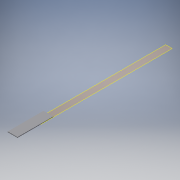
# Autodesk Inventor part: Part1
Saved by Autodesk Inventor 2016 (Build 200138000, 138)
## iProperties
Created: 2017-06-06
Part Number: Part1
Material: Generic
Document SubType Name: Modeling
Designer: m228540
Density: 1 g/cm^3
Appearance: Default
Author: m228540
Autodesk Inventor part; units mm, degrees
ref_plane "YZ Plane" through (0, 0, 0) normal (1, 0, 0) x (0, 1, 0)
ref_plane "XZ Plane" through (0, 0, 0) normal (0, 1, 0) x (-1, 0, 0)
ref_plane "XY Plane" through (0, 0, 0) normal (0, 0, 1) x (1, 0, 0)
ref_plane "Work Plane1" through (0, 0, 0) normal (0, 0, 1) x (1, 0, 0)
sketch "Sketch1" plane through (0, 0, 0) normal (0, 0, 1) x (1, 0, 0)
  line L0 (-2.396, -1045.7142) -> (-92.396, -1045.7142)
  line L1 (-92.396, -1375.7142) -> (-2.396, -1375.7142)
  line L2 (-2.396, -1375.7142) -> (-2.396, -1045.7142)
  line L3 (-92.396, -1256.8384) -> (-192.396, -1256.8384)
  line L4 (-192.396, -1256.8384) -> (-192.396, -1326.8384)
  line L5 (-192.396, -1326.8384) -> (-234.396, -1326.8384)
  line L6 (-234.396, -1326.8384) -> (-234.396, -1146.8384)
  line L7 (-182.396, -1190.8384) -> (-92.396, -1190.8384)
  line L8 (-92.396, -1045.7142) -> (-92.396, -1190.8384)
  line L9 (-92.396, -1256.8384) -> (-92.396, -1375.7142)
  line L10 (-234.396, -1146.8384) -> (-182.396, -1146.8384)
  line L11 (-182.396, -1146.8384) -> (-182.396, -1190.8384)
  point P0 (0, 0)
  dimension "d0" = 90
  dimension "d1" = 330
  dimension "d4" = 100
  dimension "d5" = 70
  dimension "d6" = 42
  dimension "d7" = 180
  dimension "d8" = 52
  dimension "d9" = 44
  constraints: 24 end point, 10 perpendicular, 3 parallel, 2 horizontal
  measures "d0" distance of L1.start L1.end
  measures "d1" distance of L0.end L1.start
  measures "d4" distance of L3.start L3.end
  measures "d5" distance of L3.end L4.end
  measures "d6" distance of L4.end L5.end
  measures "d7" distance of L5.end L6.end
  measures "d8" distance of L6.end L10.end
  measures "d9" distance of L10.end L7.start
extrude "Extrusion1" add sketch "Sketch1" along normal blind 6
body "Solid1"
